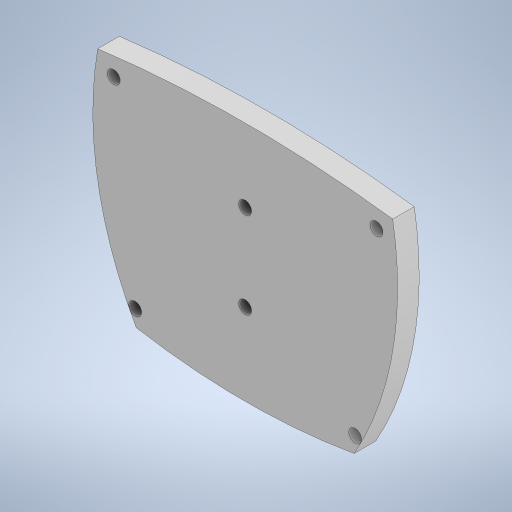
# Autodesk Inventor part: ProjEnAble_Microbit_Cover
Saved by Autodesk Inventor 2023 (Build 270158000, 158)
## iProperties
Created: 2022-11-30
Part Number: ProjEnAble_Microbit_Cover
Material: Generic
Document SubType Name: Modeling
Designer: jeron
Density: 1 g/cm^3
Appearance: Default
Author: jeron
Autodesk Inventor part; units mm, degrees
ref_plane "YZ Plane" through (0, 0, 0) normal (1, 0, 0) x (0, 1, 0)
ref_plane "XZ Plane" through (0, 0, 0) normal (0, 1, 0) x (-1, 0, 0)
ref_plane "XY Plane" through (0, 0, 0) normal (0, 0, 1) x (1, 0, 0)
sketch "Sketch1" plane through (0, 0, 0) normal (0, 0, 1) x (1, 0, 0)
  line L0 (0, 0) -> (0, 23)
  line L1 (0, 0) -> (0, -25)
  line L2 (0, 0) -> (-32.5, 0)
  line L3 (0, 0) -> (32.5, 0)
  line L4 (0, 23) -> (0, 25)
  line L5 (0, -25) -> (0, -27)
  arc A0 (32.5, 23) -> (-32.5, 23) centre (0, -240.0625) ccw
  arc A1 (-24, -25) -> (24, -25) centre (0, 118) ccw
  arc A2 (-34.2324, 24.7969) -> (-25.28, -26.8099) centre (42.3382, 11.5) ccw
  arc A3 (34.2324, 24.7969) -> (-34.2324, 24.7969) centre (0, -240.0625) ccw
  arc A4 (25.28, -26.8099) -> (34.2324, 24.7969) centre (-42.3382, 11.5) ccw
  arc A5 (-25.28, -26.8099) -> (25.28, -26.8099) centre (0, 118) ccw
  line L6 (24, -25) -> (-24, -25)
  line L7 (-32.5, 23) -> (-30.5, 23)
  line L8 (-30.5, 23) -> (-30.5, 21)
  circle A6 centre (-30.5, 21) radius 1.5
  line L9 (-27.5, 23) -> (-27.5, 18)
  line L10 (-27.5, 18) -> (-33.0989, 18)
  line L11 (-32.5, 23) -> (-30.5, 23)
  line L12 (-27.5, 23) -> (27.5, 23)
  line L13 (-27.5, 23) -> (-27.5, 23.5696)
  circle A7 centre (30.5, 21) radius 1.5
  line L14 (27.5, 23) -> (27.5, 18)
  line L15 (27.5, 18) -> (33.0989, 18)
  line L16 (27.5, 23) -> (27.5, 23.5696)
  line L17 (-25.28, -26.8099) -> (-27.252, -26.8099)
  line L18 (-27.252, -26.8099) -> (-27.2519, -23.0989)
  line L19 (-27.2519, -23.0989) -> (-25.5309, -23.099)
  circle A8 centre (-25.5309, -23.099) radius 1.5
  line L20 (-26.1342, -20.8192) -> (-24, -20.8192)
  line L21 (-24, -20.8192) -> (-24, -25)
  arc A9 (-32.5, 23) -> (-26.1342, -20.8192) centre (42.3382, 11.5) ccw
  circle A10 centre (25.5309, -23.099) radius 1.5
  line L22 (26.1342, -20.8192) -> (24, -20.8192)
  line L23 (24, -20.8192) -> (24, -25)
  arc A11 (26.1342, -20.8192) -> (32.5, 23) centre (-42.3382, 11.5) ccw
  point P0 (24, -25)
  dimension "d0" = 23
  dimension "d1" = 25
  dimension "d4" = 65
  dimension "d6" = 48
  dimension "d7" = 32.5
  dimension "d8" = 32.5
  dimension "d9" = 2
  dimension "d10" = 2
  dimension "d12" = 2
  dimension "d13" = 2
  dimension "d14" = 3
  dimension "d15" = 5
  dimension "d16" = 5
  dimension "d17" = 1.972
  dimension "d18" = 3.711
  dimension "d19" = 1.721
  dimension "d20" = 3
  constraints: 48 end point, 24 point on circle, 12 centre point, 9 symmetric about line, 7 horizontal, 5 perpendicular, 5 vertical, 2 coincident, 1 point on line, 2 other
  measures "d0" distance of L0.start L0.end
  measures "d1" distance of L0.start L1.end
  measures "d4" distance of L7.start A0.start
  measures "d6" distance of L6.start L21.end
  measures "d7" distance of L0.start L2.end
  measures "d8" distance of L0.start L3.end
  measures "d9" distance of L0.end L4.end
  measures "d10" distance of L1.end L5.end
  measures "d12" distance of L7.start L7.end
  measures "d13" distance of L7.end L8.end
  measures "d14" diameter of A6
  measures "d15" distance of L7.start L9.start
  measures "d16" distance of L9.start L9.end
  measures "d17" distance of L17.start L17.end
  measures "d18" distance of L17.end L18.end
  measures "d19" distance of L18.end L19.end
  measures "d20" diameter of A8
extrude "Extrusion1" add sketch "Sketch1" along normal blind 2 contours L2 A9 L10 L9 L12 L0 | L3 A11 L22 L23 L6 L1 | L1 L6 L21 L20 A9 L2 | L0 L12 L14 L15 A11 L3 | L12 L13 A0 L4 | L4 A0 L16 L12 | L6 A1 L5 | L5 A1 L6 | A6 | L9 L10 A9 A0 L13 | L16 A0 A11 L15 L14 | A8 | A3 A4 A5 A2 | A7 | A10
extrude "Extrusion2" add sketch "Sketch1" against normal blind 3 contours L9 L10 A9 A0 L13 | L16 A0 A11 L15 L14 | A3 A4 A5 A2
sketch "Sketch2" plane through (0, 0, 2) normal (0, 0, 1) x (1, 0, 0)
  circle A0 centre (0, 10) radius 1.5
  circle A1 centre (0, -10) radius 1.5
  point P0 (0, 0)
  dimension "d27" = 3
  dimension "d28" = 3
  constraints: 2 centre point
  measures "d27" diameter of A0
  measures "d28" diameter of A1
extrude "Extrusion3" cut sketch "Sketch2" against normal up to surface (2 mm away)
extrude "Extrusion4" cut sketch "Sketch1" along normal blind 10 contours A6 | A8 | A7 | A10
body "Solid1"
